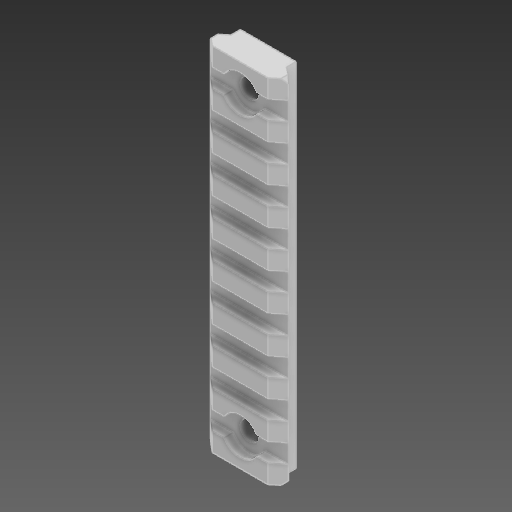
# Autodesk Inventor part: Picatinny10
Saved by Autodesk Inventor 2020.4 (Build 244396010, 396A)
## iProperties
Created: 2022-09-17
Part Number: Picatinny10
Material: Generic
Document SubType Name: Modeling
Designer: Val
Density: 1 g/cm^3
Appearance: Default
Author: Val
Autodesk Inventor part; units mm, degrees
ref_plane "YZ Plane" through (0, 0, 0) normal (1, 0, 0) x (0, 1, 0)
ref_plane "XZ Plane" through (0, 0, 0) normal (0, 1, 0) x (-1, 0, 0)
ref_plane "XY Plane" through (0, 0, 0) normal (0, 0, 1) x (1, 0, 0)
sketch "Base" plane through (0, 0, 0) normal (0, 0, 1) x (1, 0, 0)
  line L0 (-7.5, 95) -> (7.5, 95)
  line L1 (7.5, 95) -> (7.5, 0)
  line L2 (7.5, 0) -> (-7.5, 0)
  line L3 (-7.5, 0) -> (-7.5, 95)
  point P0 (0, 0)
  point P1 (0, 0)
  dimension "d0" = 95
  dimension "d1" = 15
  constraints: 8 end point, 2 parallel, 1 coincident, 1 horizontal, 1 midpoint, 1 perpendicular
  measures "d0" distance of L2.end L0.start
  measures "d1" distance of L0.start L0.end
extrude "BaseFeature" add sketch "Base" along normal blind 2.54
sketch "Profile" plane through (-7.5, 0, 0) normal (0, -1, 0) x (1, 0, 0)
  line L0 (0, 2.54) -> (15, 2.54) projected
  line L1 (0, 2.54) -> (15, 2.54)
  line L2 (15, 2.54) -> (15, 7.5692) construction
  line L3 (15, 7.5692) -> (0, 7.5692)
  line L4 (0, 7.5692) -> (0, 2.54) construction
  line L5 (-3.041, 5.0546) -> (18.041, 5.0546) construction
  line L6 (15, 7.5692) -> (18.041, 5.0546)
  line L7 (15, 2.54) -> (18.041, 5.0546)
  line L8 (0, 7.5692) -> (-3.041, 5.0546)
  line L9 (-3.041, 5.0546) -> (0, 2.54)
  point P0 (7.5, 0)
  point P1 (15, 5.0546)
  dimension "d4" = 5.0292
  dimension "d5" = 21.082
  constraints: 18 end point, 4 parallel, 2 horizontal, 1 midpoint, 1 perpendicular, 1 point on line
  measures "d4" distance of L0.end L2.end
  measures "d5" distance of L5.start L5.end
extrude "ProfileFeature" add sketch "Profile" against normal up to surface (95 mm away)
sketch "Rails" plane through (-7.5, 0, 7.5692) normal (0, 0, 1) x (1, 0, 0)
  line L0 (-3.041, 0) -> (-3.041, 95) projected
  line L1 (-3.041, 95) -> (18.041, 95)
  line L2 (18.041, 95) -> (18.041, 90)
  line L3 (18.041, 90) -> (-3.041, 90)
  line L4 (-3.041, 90) -> (-3.041, 95)
  line L5 (18.041, 0) -> (18.041, 95) projected
  line L6 (18.041, 80) -> (-3.041, 80)
  line L7 (-3.041, 85) -> (18.041, 85)
  line L8 (-3.041, 80) -> (-3.041, 85)
  line L9 (18.041, 85) -> (18.041, 80)
  line L10 (18.041, 70) -> (-3.041, 70)
  line L11 (-3.041, 75) -> (18.041, 75)
  line L12 (-3.041, 70) -> (-3.041, 75)
  line L13 (18.041, 75) -> (18.041, 70)
  line L14 (18.041, 60) -> (-3.041, 60)
  line L15 (-3.041, 65) -> (18.041, 65)
  line L16 (-3.041, 60) -> (-3.041, 65)
  line L17 (18.041, 65) -> (18.041, 60)
  line L18 (18.041, 50) -> (-3.041, 50)
  line L19 (-3.041, 55) -> (18.041, 55)
  line L20 (-3.041, 50) -> (-3.041, 55)
  line L21 (18.041, 55) -> (18.041, 50)
  line L22 (18.041, 40) -> (-3.041, 40)
  line L23 (-3.041, 45) -> (18.041, 45)
  line L24 (-3.041, 40) -> (-3.041, 45)
  line L25 (18.041, 45) -> (18.041, 40)
  line L26 (18.041, 30) -> (-3.041, 30)
  line L27 (-3.041, 35) -> (18.041, 35)
  line L28 (-3.041, 30) -> (-3.041, 35)
  line L29 (18.041, 35) -> (18.041, 30)
  line L30 (18.041, 20) -> (-3.041, 20)
  line L31 (-3.041, 25) -> (18.041, 25)
  line L32 (-3.041, 20) -> (-3.041, 25)
  line L33 (18.041, 25) -> (18.041, 20)
  line L34 (18.041, 10) -> (-3.041, 10)
  line L35 (-3.041, 15) -> (18.041, 15)
  line L36 (-3.041, 10) -> (-3.041, 15)
  line L37 (18.041, 15) -> (18.041, 10)
  line L38 (18.041, 0) -> (-3.041, 0)
  line L39 (-3.041, 5) -> (18.041, 5)
  line L40 (-3.041, 0) -> (-3.041, 5)
  line L41 (18.041, 5) -> (18.041, 0)
  point P0 (7.5, 0)
  point P1 (18.041, 0)
  point P2 (-3.041, 0)
  point P3 (18.041, 5)
  point P4 (18.041, 10)
  point P5 (-3.041, 10)
  point P6 (18.041, 15)
  point P7 (18.041, 20)
  point P8 (-3.041, 20)
  point P9 (18.041, 25)
  point P10 (18.041, 30)
  point P11 (-3.041, 30)
  point P12 (18.041, 35)
  point P13 (18.041, 40)
  point P14 (-3.041, 40)
  point P15 (18.041, 45)
  point P16 (18.041, 50)
  point P17 (-3.041, 50)
  point P18 (18.041, 55)
  point P19 (18.041, 60)
  point P20 (-3.041, 60)
  point P21 (18.041, 65)
  point P22 (18.041, 70)
  point P23 (-3.041, 70)
  point P24 (18.041, 75)
  point P25 (18.041, 80)
  point P26 (-3.041, 80)
  point P27 (18.041, 85)
  point P28 (18.041, 90)
  point P29 (-3.041, 90)
  point P30 (18.041, 95)
  dimension "d8" = 5
  dimension "d11" = 10
  constraints: 80 end point, 2 parallel, 2 vertical, 1 horizontal, 1 perpendicular, 73 other
  measures "d8" distance between parallel lines of L1 L3
  measures "d11" distance of L2.end L6.start
extrude "RailsFeature" cut sketch "Rails" against normal up to surface (2.5146 mm away) contours L0 L34 L5 L39 | L0 L30 L5 L35 | L0 L26 L5 L31 | L0 L22 L5 L27 | L0 L18 L5 L23 | L0 L14 L5 L19 | L0 L10 L5 L15 | L0 L6 L5 L11 | L0 L3 L5 L7
sketch "Corners" plane through (0, 0, 0) normal (0, 0, -1) x (-1, 0, 0)
  line L0 (-10.541, 95) -> (-7.5, 95) projected
  line L1 (-10.541, 95) -> (-9.4234, 95)
  line L2 (-9.4234, 95) -> (-9.4234, 93.8824)
  line L3 (-9.4234, 93.8824) -> (-10.541, 93.8824)
  line L4 (-10.541, 93.8824) -> (-10.541, 95)
  line L5 (0, -19) -> (0, 114) construction
  line L6 (10.541, 95) -> (9.4234, 95)
  line L7 (9.4234, 95) -> (9.4234, 93.8824)
  line L8 (9.4234, 93.8824) -> (10.541, 93.8824)
  line L9 (10.541, 93.8824) -> (10.541, 95)
  line L10 (-7.5, 95) -> (7.5, 95) construction
  line L11 (0, 95) -> (0, 0) construction
  line L12 (0, 47.5) -> (10.541, 47.5) construction
  line L13 (-10.541, 0) -> (-9.4234, 0)
  line L14 (-9.4234, 0) -> (-9.4234, 1.1176)
  line L15 (-9.4234, 1.1176) -> (-10.541, 1.1176)
  line L16 (-10.541, 1.1176) -> (-10.541, 0)
  line L17 (10.541, 0) -> (9.4234, 0)
  line L18 (10.541, 1.1176) -> (10.541, 0)
  line L19 (9.4234, 0) -> (9.4234, 1.1176)
  line L20 (9.4234, 1.1176) -> (10.541, 1.1176)
  line L21 (-10.541, 93.8824) -> (-9.4234, 95)
  line L22 (9.4234, 95) -> (10.541, 93.8824)
  line L23 (9.4234, 0) -> (10.541, 1.1176)
  line L24 (-10.541, 1.1176) -> (-9.4234, 0)
  dimension "d36" = 1.1176
  constraints: 44 end point, 12 symmetric about line, 6 perpendicular, 2 horizontal, 2 midpoint, 2 parallel
  measures "d36" distance of L2.end L3.end
extrude "CornersFeature" cut sketch "Corners" against normal through all contours L0 L21 L4 | L9 L22 L6 | L16 L24 L13 | L17 L23 L18
sketch "MountHoles" plane through (-10.541, 80, 5.0546) normal (0, 0, 1) x (1, 0, 0)
  line L0 (0, 0) -> (21.082, 0) construction
  line L1 (0, -5) -> (0, 0) construction
  line L2 (21.082, -5) -> (0, -5) construction
  line L3 (21.082, -5) -> (21.082, 0) construction
  line L4 (0, -75) -> (0, -70) construction
  line L5 (21.082, 5) -> (21.082, 10) construction
  line L6 (0, -10) -> (21.082, -10) projected
  line L7 (0, -15) -> (0, -10) projected
  line L8 (21.082, -15) -> (0, -15) projected
  line L9 (21.082, -15) -> (21.082, -10) projected
  line L10 (0, -50) -> (21.082, -50) projected
  line L11 (0, -55) -> (0, -50) projected
  line L12 (21.082, -55) -> (0, -55) projected
  line L13 (21.082, -55) -> (21.082, -50) projected
  line L14 (0, -60) -> (21.082, -60) projected
  line L15 (0, -65) -> (0, -60) projected
  line L16 (21.082, -65) -> (0, -65) projected
  line L17 (21.082, -65) -> (21.082, -60) projected
  line L18 (0, -20) -> (21.082, -20) projected
  line L19 (0, -25) -> (0, -20) projected
  line L20 (21.082, -25) -> (0, -25) projected
  line L21 (21.082, -25) -> (21.082, -20) projected
  line L22 (0, 0) -> (21.082, 0) projected
  line L23 (0, -5) -> (0, 0) projected
  line L24 (21.082, -5) -> (0, -5) projected
  line L25 (21.082, -5) -> (21.082, 0) projected
  line L26 (0, -40) -> (21.082, -40) projected
  line L27 (0, -45) -> (0, -40) projected
  line L28 (21.082, -45) -> (0, -45) projected
  line L29 (21.082, -45) -> (21.082, -40) projected
  line L30 (0, -70) -> (21.082, -70) projected
  line L31 (21.082, -75) -> (0, -75) projected
  line L32 (21.082, -75) -> (21.082, -70) projected
  line L33 (0, -30) -> (21.082, -30) projected
  line L34 (0, -35) -> (0, -30) projected
  line L35 (21.082, -35) -> (0, -35) projected
  line L36 (21.082, -35) -> (21.082, -30) projected
  line L37 (0, 10) -> (21.082, 10) projected
  line L38 (0, 5) -> (0, 10) projected
  line L39 (21.082, 5) -> (0, 5) projected
  circle A0 centre (10.541, 7.5) radius 2.5
  circle A1 centre (10.541, -72.5) radius 2.5
  line L40 (3.041, -70) -> (18.041, -70) projected
  line L41 (18.041, -75) -> (3.041, -75) projected
  line L42 (3.041, 10) -> (18.041, 10) projected
  line L43 (18.041, 5) -> (3.041, 5) projected
  line L44 (18.041, 15) -> (3.041, 15) projected
  line L45 (10.541, 15) -> (10.541, -80) construction
  line L46 (18.041, -80) -> (3.041, -80) projected
  constraints: 6 tangent, 2 centre point, 2 end point, 2 midpoint, 2 point on line
hole "MountHolesFeature" at (0, 87.5, 5.0546) at (0, 7.5, 5.0546) direction (0, 0, -1) diameter 5 depth 25.4 tip angle 118
sketch "Countersinks" plane through (-10.541, 15, 5.0546) normal (0, 0, 1) x (1, 0, 0)
  arc A0 (10.541, 70) -> (10.541, 75) centre (10.541, 72.5) ccw construction
  arc A1 (10.541, -10) -> (10.541, -5) centre (10.541, -7.5) ccw construction
  circle A2 centre (10.541, 72.5) radius 5
  circle A3 centre (10.541, -7.5) radius 5
  dimension "d39" = 10
  constraints: 2 centre point, 2 coincident, 1 equal radius
  measures "d39" diameter of A2
extrude "CountersinksFeature" cut sketch "Countersinks" along normal through all
sketch "Spacers" plane through (0, 0, 0) normal (0, 0, -1) x (-1, 0, 0)
  circle A0 centre (0, 87.5) radius 2.5 projected
  circle A1 centre (0, 7.5) radius 2.5 projected
  circle A2 centre (0, 87.5) radius 4.5
  circle A3 centre (0, 7.5) radius 4.5
  point P0 (0, 117.5)
  dimension "d40" = 2
  constraints: 2 centre point, 2 coincident, 1 equal radius
  measures "d40" radial gap between concentric circles of A2 A0
extrude "SpacersFeature" add sketch "Spacers" along normal blind 1
body "Solid1"
